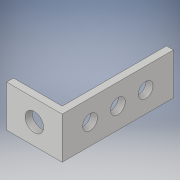
# Autodesk Inventor part: simpleBracketForTopOfDart
Saved by Autodesk Inventor 2017 (Build 210142000, 142)
## iProperties
Created: 2016-05-06
Part Number: simpleBracketForTopOfDart
Material: Generic
Document SubType Name: Modeling
Designer: steele
Density: 1 g/cm^3
Appearance: Default
Author: steele
Autodesk Inventor part; units mm, degrees
ref_plane "YZ Plane" through (0, 0, 0) normal (1, 0, 0) x (0, 1, 0)
ref_plane "XZ Plane" through (0, 0, 0) normal (0, 1, 0) x (-1, 0, 0)
ref_plane "XY Plane" through (0, 0, 0) normal (0, 0, 1) x (1, 0, 0)
sketch "Sketch1" plane through (0, 0, 0) normal (0, 1, 0) x (-1, 0, 0)
  line L0 (0, 0) -> (25.4, 0)
  line L1 (25.4, 0) -> (25.4, -3.175)
  line L2 (25.4, -3.175) -> (3.175, -3.175)
  line L3 (3.175, -3.175) -> (3.175, -50.8)
  line L4 (3.175, -50.8) -> (0, -50.8)
  line L5 (0, -50.8) -> (0, 0)
  dimension "d0" = 25.4
  dimension "d1" = 50.8
  dimension "d2" = 3.175
  dimension "d3" = 3.175
  constraints: 12 end point, 5 perpendicular, 1 horizontal
  measures "d0" distance of L0.start L0.end
  measures "d1" distance of L4.end L0.start
  measures "d2" distance between parallel lines of L2 L0
  measures "d3" distance between parallel lines of L3 L5
extrude "Extrusion1" add sketch "Sketch1" along normal mid plane 18.9992
sketch "Sketch2" plane through (-25.4, 9.4996, 0) normal (0, 0, 1) x (1, 0, 0)
  line L0 (0, 0) -> (25.4, 0) construction
  line L1 (25.4, -18.9992) -> (25.4, 0) construction
  line L2 (0, 0) -> (25.4, -18.9992) construction
  line L3 (0, 0) -> (0, -18.9992) construction
  line L4 (0, -18.9992) -> (25.4, 0) construction
  point P0 (25.4, -9.4996)
  point P1 (12.7, -9.4996)
  constraints: 4 end point, 1 midpoint
hole "Hole1" at (-12.7, 0, 0) direction (0, 0, -1) diameter 8.4328 end through all clearance for "Flat Head Machine Screw (82)" size "5/16" standard "Ansi Unified Screw Threads"
sketch "Sketch3" plane through (0, -9.4996, -50.8) normal (1, 0, 0) x (0, 0, -1)
  line L0 (0, 18.9992) -> (0, 0) construction
  line L1 (-50.8, 18.9992) -> (-50.8, 0) construction
  line L2 (0, 0) -> (-50.8, 0) construction
  line L3 (-50.8, 9.4996) -> (0, 9.4996) construction
  point P0 (-38.1, 9.4996)
  point P1 (-25.4, 9.4996)
  point P2 (-12.7, 9.4996)
  dimension "d20" = 12.7
  dimension "d23" = 12.7
  constraints: 2 end point, 1 horizontal, 1 midpoint, 1 point on line, 2 other
  measures "d20" distance from line of point (-38.1, 9.5) L1
  measures "d23" distance of point (-38.1, 9.5) point (-25.4, 9.5)
hole "Hole3" at (0, 0, -12.7) at (0, 0, -25.4) at (0, 0, -38.1) direction (-1, 0, 0) diameter 6.7564 end through all clearance for "Flat Head Machine Screw (82)" size "1/4" standard "Ansi Unified Screw Threads"
body "Solid1"
